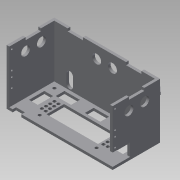
# Autodesk Inventor part: Kepala Belakang 2
Saved by Autodesk Inventor 2015 SP1 (Build 190203100, 203)
## iProperties
Created: 2015-02-01
Part Number: Kepala Belakang 2
Material: Generic
Document SubType Name: Modeling
Designer: Rafi Kurnia Putra
Density: 1 g/cm^3
Appearance: Default
Mass: 66.641 g
Surface Area: 406.742 cm^2
Volume: 66.641 cm^3
Author: Rafi Kurnia Putra
Autodesk Inventor part; units mm, degrees
(part 1 of 2)
ref_plane "YZ Plane" through (0, 0, 0) normal (1, 0, 0) x (0, 1, 0)
ref_plane "XY Plane" through (0, 0, 0) normal (0, 0, 1) x (1, 0, 0)
sketch "Sketch1" plane through (0, 0, 0) normal (0, 1, 0) x (-1, 0, 0)
  line L0 (60.406, -27.1071) -> (-60.406, -27.1071)
  line L1 (-60.406, -27.1071) -> (-60.406, 27.1071)
  line L2 (-60.406, 27.1071) -> (60.406, 27.1071)
  line L3 (60.406, 27.1071) -> (60.406, -27.1071)
  line L4 (60.406, -27.1071) -> (-60.406, 27.1071) construction
  line L5 (-60.406, -27.1071) -> (60.406, 27.1071) construction
  line L6 (-57.406, 24.1071) -> (-57.406, -27.1071)
  line L7 (57.406, -27.1071) -> (57.406, 24.1071)
  line L8 (57.406, 24.1071) -> (-57.406, 24.1071)
  point P0 (0, 0)
  point P1 (0, 0)
  dimension "d49" = 120.812
  dimension "d51" = 3
  dimension "d57" = 3
  dimension "d58" = 3
  dimension "d59" = 114.812
  dimension "d61" = 51.2141
  constraints: 18 end point, 3 midpoint, 3 parallel, 2 point on line, 1 horizontal, 1 perpendicular, 1 other
  measures "d49" distance of L1.end L2.end
  measures "d51" distance between parallel lines of L6 L1
  measures "d57" distance between parallel lines of L7 L3
  measures "d58" distance between parallel lines of L8 L2
  measures "d59" distance between parallel lines of L7 L6
  measures "d61" distance between parallel lines of L8 L0
extrude "Extrusion5" add sketch "Sketch1" against normal blind 3
extrude "Extrusion6" add sketch "Sketch1" along normal blind 60 contours L0 L7 L8 L6 L1 L2 L3
sketch "Sketch6" plane through (0, -3, 0) normal (0, -1, 0) x (1, 0, 0)
  circle A0 centre (-50.5965, 17.5471) radius 1.75
  circle A1 centre (50.5965, 17.5471) radius 1
  circle A2 centre (50.5965, 17.5471) radius 1.75
  circle A3 centre (-50.5965, 17.5471) radius 1.75
  point P0 (0, 0)
  dimension "d62" = 3.5
  constraints: 4 centre point, 2 coincident, 1 concentric, 4 other
  measures "d62" diameter of A2
extrude "Extrusion7" cut sketch "Sketch6" against normal up to next contours A0 | A1 | A2
sketch "Sketch7" plane through (0, -3, 0) normal (0, -1, 0) x (1, 0, 0)
  line L0 (-53.556, -8.4641) -> (-43.556, -8.4641)
  line L1 (-43.556, -8.4641) -> (-43.556, 9.0359)
  line L2 (-43.556, 9.0359) -> (-53.556, 9.0359)
  line L3 (-53.556, 9.0359) -> (-53.556, -8.4641)
  line L4 (-53.556, -8.4641) -> (-43.556, 9.0359) construction
  line L5 (-43.556, -8.4641) -> (-53.556, 9.0359) construction
  line L6 (53.556, -8.4641) -> (43.556, -8.4641)
  line L7 (43.556, -8.4641) -> (43.556, 9.0359)
  line L8 (43.556, 9.0359) -> (53.556, 9.0359)
  line L9 (53.556, 9.0359) -> (53.556, -8.4641)
  line L10 (53.556, -8.4641) -> (43.556, 9.0359) construction
  line L11 (43.556, -8.4641) -> (53.556, 9.0359) construction
  line L12 (-42.0848, 10.5071) -> (-24.5848, 10.5071)
  line L13 (-24.5848, 10.5071) -> (-24.5848, 20.5071)
  line L14 (-24.5848, 20.5071) -> (-42.0848, 20.5071)
  line L15 (-42.0848, 20.5071) -> (-42.0848, 10.5071)
  line L16 (-42.0848, 10.5071) -> (-24.5848, 20.5071) construction
  line L17 (-24.5848, 10.5071) -> (-42.0848, 20.5071) construction
  line L18 (42.0848, 10.5071) -> (24.5848, 10.5071)
  line L19 (24.5848, 10.5071) -> (24.5848, 20.5071)
  line L20 (24.5848, 20.5071) -> (42.0848, 20.5071)
  line L21 (42.0848, 20.5071) -> (42.0848, 10.5071)
  line L22 (42.0848, 10.5071) -> (24.5848, 20.5071) construction
  line L23 (24.5848, 10.5071) -> (42.0848, 20.5071) construction
  point P0 (0, 0)
  point P1 (-48.556, 0.2859)
  point P2 (-48.556, 0.2859)
  point P3 (48.556, 0.2859)
  point P4 (48.556, 0.2859)
  point P5 (-33.3348, 15.5071)
  point P6 (-33.3348, 15.5071)
  point P7 (33.3348, 15.5071)
  point P8 (33.3348, 15.5071)
  dimension "d65" = 10
  dimension "d66" = 17.5
  dimension "d69" = 10
  constraints: 48 end point, 10 midpoint, 4 parallel, 2 horizontal, 2 perpendicular
  measures "d65" distance of L2.end L1.end
  measures "d66" distance of L1.end L0.end
  measures "d69" distance of L13.end L12.end
extrude "Extrusion8" cut sketch "Sketch7" against normal up to next
sketch "Sketch9" plane through (0, 60, 0) normal (0, 1, 0) x (1, 0, 0)
  line L0 (60.406, 8.4641) -> (56.906, 8.4641)
  line L1 (56.906, -9.0359) -> (60.406, -9.0359)
  line L2 (60.406, 8.4641) -> (60.406, -9.0359)
  line L3 (56.906, -9.0359) -> (56.906, 8.4641)
  line L4 (42.0848, -23.8571) -> (42.0848, -27.3571)
  line L5 (42.0848, -27.3571) -> (24.5848, -27.3571)
  line L6 (24.5848, -23.8571) -> (42.0848, -23.8571)
  line L7 (24.5848, -23.8571) -> (24.5848, -27.3571)
  line L8 (0, 0) -> (0, -13)
  line L9 (-60.406, 8.4641) -> (-56.906, 8.4641)
  line L10 (-56.906, -9.0359) -> (-60.406, -9.0359)
  line L11 (-60.406, 8.4641) -> (-60.406, -9.0359)
  line L12 (-56.906, -9.0359) -> (-56.906, 8.4641)
  line L13 (-42.0848, -23.8571) -> (-42.0848, -27.3571)
  line L14 (-42.0848, -27.3571) -> (-24.5848, -27.3571)
  line L15 (-24.5848, -23.8571) -> (-42.0848, -23.8571)
  line L16 (-24.5848, -23.8571) -> (-24.5848, -27.3571)
  constraints: 34 end point, 8 symmetric about line, 2 vertical, 1 horizontal, 1 parallel
extrude "Extrusion9" cut sketch "Sketch9" against normal blind 3
sketch "Sketch10" plane through (0, -3, 0) normal (0, -1, 0) x (1, 0, 0)
  circle A0 centre (-32.4485, -17.4559) radius 1.75
  circle A1 centre (-37.593, 4.5441) radius 1.75
  circle A2 centre (32.4355, -17.4559) radius 1.75
  circle A3 centre (37.593, 4.5441) radius 1.75
  point P0 (0, 0)
  dimension "d84" = 22
  dimension "d85" = 22
  constraints: 4 centre point, 4 other
  measures "d84" vertical distance of A1.centre A0.centre
  measures "d85" vertical distance of A3.centre A2.centre
extrude "Extrusion10" cut sketch "Sketch10" against normal up to next
sketch "Sketch12" plane through (-60.406, -3, -27.1071) normal (-1, 0, 0) x (0, 0, 1)
  circle A0 centre (3, 59.0338) radius 1
  circle A1 centre (3, 38.0338) radius 1
  arc A2 (6.0857, 8.75) -> (6.7857, 8.05) centre (6.7857, 8.75) ccw
  arc A3 (13.0857, 8.05) -> (13.7857, 8.75) centre (13.0857, 8.75) ccw
  line L0 (13.0857, 8.05) -> (6.7857, 8.05)
  arc A4 (7.3007, 11.65) -> (6.9007, 11.25) centre (7.3007, 11.25) ccw
  arc A5 (12.9707, 11.25) -> (12.5707, 11.65) centre (12.5707, 11.25) ccw
  line L1 (7.3007, 11.25) -> (13.0857, 8.75) construction
  line L2 (13.0857, 8.75) -> (6.7857, 8.75) construction
  line L3 (6.7857, 8.75) -> (12.5707, 11.25) construction
  line L4 (2.4357, 5.1113) -> (17.4357, 5.1113)
  line L5 (17.4357, 5.1113) -> (17.4357, 15.1113)
  line L6 (17.4357, 15.1113) -> (2.4357, 15.1113)
  line L7 (2.4357, 15.1113) -> (2.4357, 5.1113)
  line L8 (2.4357, 5.1113) -> (17.4357, 15.1113) construction
  line L9 (17.4357, 5.1113) -> (2.4357, 15.1113) construction
  point P0 (27.1071, 3)
  point P1 (9.9357, 10.1113)
  dimension "d86" = 15
  dimension "d87" = 10
  constraints: 20 end point, 8 point on circle, 6 centre point, 3 horizontal, 2 midpoint, 2 parallel, 2 point on line, 1 perpendicular, 20 other
  measures "d86" distance of L6.end L5.end
  measures "d87" distance of L5.end L4.end
extrude "Extrusion11" cut sketch "Sketch12" against normal blind 200 contours A0 | A1
extrude "Extrusion12" cut sketch "Sketch12" against normal up to next contours L7 L6 L5 L4
fillet "Fillet2" radius 2 4 edges at (-58.906, 12.1113, -24.6713) (-58.906, 12.1113, -9.6713) (-58.906, 2.1113, -24.6713) (-58.906, 2.1113, -9.6713)
sketch "Sketch13" plane through (0, -3, 0) normal (0, -1, 0) x (1, 0, 0)
  line L0 (29.3575, 1.3171) -> (-29.3575, 1.3171)
  circle A0 centre (-32.8575, 4.3056) radius 1.75
  circle A1 centre (32.8575, 4.3056) radius 1.75
  line L1 (29.3575, 1.3171) -> (29.3575, 7.2941)
  line L2 (-29.3575, 1.3171) -> (-29.3575, 7.2941)
  line L3 (-29.3575, 7.2941) -> (29.3575, 7.2941)
  line L4 (-16, -57.1829) -> (-36, -57.1829)
  line L5 (-36, -57.1829) -> (-36, -2.1829)
  line L6 (-36, -2.1829) -> (-16, -2.1829)
  line L7 (-16, -2.1829) -> (-16, -57.1829)
  line L8 (-16, -57.1829) -> (-36, -2.1829) construction
  line L9 (-36, -57.1829) -> (-16, -2.1829) construction
  point P0 (0, 0)
  point P1 (34.6075, 4.3056)
  point P2 (29.3575, 4.3056)
  point P3 (-26, -29.6829)
  dimension "d96" = 3.5
  dimension "d95" = 3.5
  dimension "d97" = 3.5
  dimension "d99" = 20
  dimension "d100" = 55
  dimension "d101" = 3.5
  constraints: 20 end point, 3 horizontal, 3 perpendicular, 2 midpoint, 2 parallel, 1 centre point, 1 horizontal alignment, 3 other
  measures "d95" diameter of A0
  measures "d97" distance of point (32.857, 4.306) point (29.357, 4.306)
  measures "d99" distance of L5.end L6.end
  measures "d100" distance of L4.end L5.end
  measures "d101" distance between parallel lines of L0 L6
extrude "Extrusion13" cut sketch "Sketch13" against normal up to next contours L0 L2 L3 L1 | A0 | A1
ref_plane "Work Plane1" through (0, 19.75, 0) normal (0, 1, 0) x (-1, 0, 0)
sketch "Sketch20" plane through (-60.406, -3, -27.1071) normal (-1, 0, 0) x (0, 0, 1)
  line L0 (30.5999, 17.25) -> (30.5999, 19.25) projected
  arc A0 (31.0999, 19.75) -> (30.5999, 19.25) centre (31.0999, 19.25) ccw projected
  line L1 (31.0999, 19.75) -> (32.0999, 19.75) projected
  arc A1 (32.5999, 19.25) -> (32.0999, 19.75) centre (32.0999, 19.25) ccw projected
  line L2 (32.5999, 19.25) -> (32.5999, 17.25) projected
  line L3 (32.0999, 16.75) -> (31.0999, 16.75) projected
  arc A2 (30.5999, 17.25) -> (31.0999, 16.75) centre (31.0999, 17.25) ccw projected
  circle A3 centre (25.0999, 18.25) radius 3.75 projected
  arc A4 (32.0999, 16.75) -> (32.5999, 17.25) centre (32.0999, 17.25) ccw projected
  line L4 (31.0999, 19.25) -> (32.0999, 17.25) construction
  line L5 (32.0999, 17.25) -> (32.0999, 19.25) construction
  line L6 (30.5999, 19.25) -> (30.5999, 17.25) construction
  line L7 (32.0999, 19.25) -> (31.0999, 17.25) construction
  point P0 (27.1071, 3)
  point P1 (31.5999, 18.25)
  dimension "d132" = 6.5
  constraints: 6 end point, 1 midpoint, 1 parallel
  measures "d132" distance of point (31.6, 18.25) A3.centre
sketch "Sketch22" plane through (60.406, -3, 27.1071) normal (1, 0, 0) x (0, 0, -1)
  circle A0 centre (35.5712, 49.2838) radius 5.125
  circle A1 centre (17.5712, 49.2838) radius 5.125
  point P0 (27.1071, 3)
  point P1 (26.5712, 49.2838)
  dimension "d246" = 10.25
  dimension "d247" = 10.25
  dimension "d248" = 18
  dimension "d249" = 9
  constraints: 2 centre point, 1 other
  measures "d246" diameter of A0
  measures "d247" diameter of A1
  measures "d248" distance of A0.centre A1.centre
  measures "d249" distance of point (26.571, 49.284) A1.centre
sketch "Sketch23" plane through (-60.406, -3, 27.1071) normal (0, 0, 1) x (1, 0, 0)
  circle A0 centre (69.406, 49.2838) radius 5.125
  circle A1 centre (51.406, 49.2838) radius 5.125
  point P0 (60.406, 3)
  point P1 (60.406, 49.2838)
  dimension "d240" = 10.25
  dimension "d241" = 10.25
  dimension "d242" = 18
  dimension "d243" = 9
  constraints: 2 centre point, 1 other
  measures "d240" diameter of A0
  measures "d241" diameter of A1
  measures "d242" distance of A0.centre A1.centre
  measures "d243" distance of point (60.406, 49.284) A1.centre
sketch "Sketch24" plane through (0, -3, 0) normal (0, -1, 0) x (1, 0, 0)
  line L0 (53.556, -27.1071) -> (53.556, -43.2141)
  line L1 (43.556, -43.2141) -> (43.556, -27.1071)
  line L2 (53.556, -43.2141) -> (43.556, -43.2141)
  line L3 (53.556, -43.2141) -> (53.556, -23.2141)
  line L4 (53.556, -23.2141) -> (43.556, -23.2141)
  line L5 (43.556, -23.2141) -> (43.556, -27.1071)
  point P0 (0, 0)
  dimension "d164" = 20
  constraints: 12 end point, 3 vertical, 2 perpendicular, 1 horizontal, 4 other
  measures "d164" distance of L0.end L3.end
extrude "Extrusion26" cut sketch "Sketch24" against normal up to next
sketch "Sketch25" plane through (-60.406, -3, 27.1071) normal (0, 0, 1) x (1, 0, 0)
  line L0 (120.812, 22) -> (120.812, 14.5) projected
  line L1 (0, 63) -> (0, 0) projected
  line L2 (120.812, 18.25) -> (241.624, 18.25) construction
  circle A0 centre (41.322, 40.0298) radius 1.6 projected
  line L3 (41.322, 40.0298) -> (41.322, 18.25)
  circle A1 centre (79.49, 40.0298) radius 1.6 projected
  line L4 (79.49, 40.0298) -> (79.49, 18.25)
  line L5 (120.812, 18.25) -> (79.49, 18.25)
  line L6 (41.322, 18.25) -> (0, 18.25)
  arc A2 (103.901, 18.25) -> (96.401, 18.25) centre (100.151, 18.25) ccw
  arc A3 (24.411, 18.25) -> (16.911, 18.25) centre (20.661, 18.25) ccw
  arc A4 (16.911, 8) -> (24.411, 8) centre (20.661, 8) ccw
  arc A5 (96.401, 8) -> (103.901, 8) centre (100.151, 8) ccw
  line L7 (3, 3) -> (117.812, 3) projected
  line L8 (16.911, 18.25) -> (16.911, 8)
  line L9 (24.411, 18.25) -> (24.411, 8)
  line L10 (96.401, 18.25) -> (96.401, 8)
  line L11 (103.901, 18.25) -> (103.901, 8)
  point P0 (60.406, 3)
  dimension "d168" = 7.5
  dimension "d169" = 7.5
  dimension "d257" = 7.5
  dimension "d258" = 7.5
  dimension "d259" = 5
  dimension "d260" = 5
  constraints: 18 end point, 8 point on circle, 4 centre point, 4 perpendicular, 4 point on line, 4 tangent, 3 midpoint, 1 horizontal, 1 parallel
  measures "d168" diameter of A2
  measures "d169" diameter of A3
  measures "d257" diameter of A4
  measures "d258" diameter of A5
  measures "d259" distance from line of A4.centre L7
  measures "d260" distance from line of A5.centre L7
sketch "Sketch26" plane through (-60.406, -3, 27.1071) normal (0, 0, 1) x (1, 0, 0)
  circle A0 centre (20.661, 18.25) radius 3.75 projected
  circle A1 centre (100.151, 18.25) radius 3.75 projected
  line L0 (9.411, 40.5) -> (31.911, 40.5)
  line L1 (31.911, 40.5) -> (31.911, 37.5)
  line L2 (31.911, 37.5) -> (9.411, 37.5)
  line L3 (9.411, 37.5) -> (9.411, 40.5)
  line L4 (9.411, 40.5) -> (31.911, 37.5) construction
  line L5 (31.911, 40.5) -> (9.411, 37.5) construction
  line L6 (88.901, 40.5) -> (111.401, 40.5)
  line L7 (111.401, 40.5) -> (111.401, 37.5)
  line L8 (111.401, 37.5) -> (88.901, 37.5)
  line L9 (88.901, 37.5) -> (88.901, 40.5)
  line L10 (88.901, 40.5) -> (111.401, 37.5) construction
  line L11 (111.401, 40.5) -> (88.901, 37.5) construction
  line L12 (120.812, 0) -> (0, 0) projected
  point P0 (60.406, 3)
  point P1 (20.661, 39)
  point P2 (100.151, 39)
  dimension "d172" = 22.5
  dimension "d173" = 3
  dimension "d174" = 22.5
  dimension "d254" = 37.5
  dimension "d255" = 37.5
  dimension "d256" = 79.49
  constraints: 24 end point, 4 midpoint, 4 parallel, 2 horizontal, 2 perpendicular
  measures "d172" distance of L1.end L2.end
  measures "d173" distance of L0.end L1.end
  measures "d174" distance of L7.end L8.end
  measures "d254" distance between parallel lines of L12 L2
  measures "d255" distance between parallel lines of L12 L8
  measures "d256" distance of point (100.151, 39) point (20.661, 39)
extrude "Extrusion28" add sketch "Sketch26" along normal blind 15 contours L0 L1 L2 L3 | L6 L7 L8 L9
sketch "Sketch27" plane through (-50.995, 37.5, 27.1071) normal (0, 1, 0) x (1, 0, 0)
  circle A0 centre (-13.5951, 23.8524) radius 3.75 projected
  line L0 (0, 0) -> (22.5, 0) projected
  line L1 (0, 0) -> (0, -15) projected
  line L2 (22.5, -15) -> (0, -15) projected
  line L3 (22.5, 0) -> (22.5, -15) projected
  line L4 (79.49, 0) -> (101.99, 0) projected
  line L5 (79.49, 0) -> (79.49, -15) projected
  line L6 (101.99, -15) -> (79.49, -15) projected
  line L7 (101.99, 0) -> (101.99, -15) projected
  circle A1 centre (11.25, -7.5) radius 3.75
  circle A2 centre (90.74, -7.5) radius 3.75
  point P0 (50.995, 27.1071)
  dimension "d177" = 7.5
  dimension "d178" = 7.5
  constraints: 2 centre point
  measures "d177" diameter of A1
  measures "d178" diameter of A2
extrude "Extrusion29" cut sketch "Sketch27" against normal up to next contours A1 | A2
sketch "Sketch30" plane through (28.495, 37.5, 27.1071) normal (0, 1, 0) x (1, 0, 0)
  circle A0 centre (-68.24, -7.5) radius 3.75 projected
  circle A1 centre (11.25, -7.5) radius 3.75 projected
  line L0 (17.25, -9) -> (18.25, -9)
  line L1 (18.75, -8.5) -> (18.75, -6.5)
  line L2 (18.25, -6) -> (17.25, -6)
  line L3 (16.75, -6.5) -> (16.75, -8.5)
  line L4 (16.75, -9) -> (18.75, -6) construction
  line L5 (18.75, -9) -> (16.75, -6) construction
  line L6 (4.25, -9) -> (5.25, -9)
  line L7 (5.75, -8.5) -> (5.75, -6.5)
  line L8 (5.25, -6) -> (4.25, -6)
  line L9 (3.75, -6.5) -> (3.75, -8.5)
  line L10 (3.75, -9) -> (5.75, -6) construction
  line L11 (5.75, -9) -> (3.75, -6) construction
  line L12 (-62.24, -9) -> (-61.24, -9)
  line L13 (-60.74, -8.5) -> (-60.74, -6.5)
  line L14 (-61.24, -6) -> (-62.24, -6)
  line L15 (-62.74, -6.5) -> (-62.74, -8.5)
  line L16 (-62.74, -9) -> (-60.74, -6) construction
  line L17 (-60.74, -9) -> (-62.74, -6) construction
  line L18 (-74.24, -9) -> (-75.24, -9)
  line L19 (-75.74, -8.5) -> (-75.74, -6.5)
  line L20 (-75.24, -6) -> (-74.24, -6)
  line L21 (-73.74, -6.5) -> (-73.74, -8.5)
  line L22 (-73.74, -9) -> (-75.74, -6) construction
  line L23 (-75.74, -9) -> (-73.74, -6) construction
  arc A2 (-75.24, -6) -> (-75.74, -6.5) centre (-75.24, -6.5) ccw
  arc A3 (-73.74, -6.5) -> (-74.24, -6) centre (-74.24, -6.5) ccw
  arc A4 (-74.24, -9) -> (-73.74, -8.5) centre (-74.24, -8.5) ccw
  arc A5 (-75.74, -8.5) -> (-75.24, -9) centre (-75.24, -8.5) ccw
  arc A6 (-61.24, -9) -> (-60.74, -8.5) centre (-61.24, -8.5) ccw
  arc A7 (-60.74, -6.5) -> (-61.24, -6) centre (-61.24, -6.5) ccw
  arc A8 (-62.24, -6) -> (-62.74, -6.5) centre (-62.24, -6.5) ccw
  arc A9 (-62.74, -8.5) -> (-62.24, -9) centre (-62.24, -8.5) ccw
  arc A10 (16.75, -8.5) -> (17.25, -9) centre (17.25, -8.5) ccw
  arc A11 (17.25, -6) -> (16.75, -6.5) centre (17.25, -6.5) ccw
  arc A12 (18.75, -6.5) -> (18.25, -6) centre (18.25, -6.5) ccw
  arc A13 (18.25, -9) -> (18.75, -8.5) centre (18.25, -8.5) ccw
  arc A14 (5.25, -9) -> (5.75, -8.5) centre (5.25, -8.5) ccw
  arc A15 (5.75, -6.5) -> (5.25, -6) centre (5.25, -6.5) ccw
  arc A16 (4.25, -6) -> (3.75, -6.5) centre (4.25, -6.5) ccw
  arc A17 (3.75, -8.5) -> (4.25, -9) centre (4.25, -8.5) ccw
  point P0 (-28.495, 27.1071)
  point P1 (17.75, -7.5)
  point P2 (4.75, -7.5)
  point P3 (-61.74, -7.5)
  point P4 (-74.74, -7.5)
  dimension "d187" = 2
  dimension "d188" = 3
  dimension "d189" = 6.5
  dimension "d190" = 2
  dimension "d191" = 3
  dimension "d192" = 6.5
  dimension "d193" = 2
  dimension "d194" = 3
  dimension "d195" = 2
  dimension "d196" = 3
  dimension "d197" = 6.5
  dimension "d198" = 6.5
  dimension "d199" = 0.5
  constraints: 48 end point, 32 point on circle, 32 point on line, 32 tangent, 16 centre point, 15 equal radius, 8 midpoint, 8 parallel, 4 horizontal, 4 perpendicular
  measures "d187" distance of L5.end L4.end
  measures "d188" distance of L4.end L5.start
  measures "d189" distance of point (17.75, -7.5) A1.centre
  measures "d190" distance of L11.end L10.end
  measures "d191" distance of L10.end L11.start
  measures "d192" distance of point (4.75, -7.5) A1.centre
  measures "d193" distance of L17.end L16.end
  measures "d194" distance of L16.end L17.start
  measures "d195" distance of L22.end L23.end
  measures "d196" distance of L23.start L22.end
  measures "d197" distance of point (-74.74, -7.5) A0.centre
  measures "d198" distance of A0.centre point (-61.74, -7.5)
  measures "d199" radius of A2
extrude "Extrusion30" cut sketch "Sketch30" against normal up to next contours A10 L3 A11 L2 A12 L1 A13 L0 | A17 L9 A16 L8 A15 L7 A14 L6 | A9 L15 A8 L14 A7 L13 A6 L12 | L18 A5 L19 A2 L20 A3 L21 A4
chamfer "Chamfer1" distance 5 angle 45 4 edges at (-50.995, 36, 42.1071) (-28.495, 36, 42.1071) (28.495, 36, 42.1071) (50.995, 36, 42.1071)
sketch "Sketch34" plane through (-60.406, -3, -27.1071) normal (-1, 0, 0) x (0, 0, 1)
  line L0 (17.4357, 13.1113) -> (17.4357, 7.1113) projected
  arc A0 (15.4357, 5.1113) -> (17.4357, 7.1113) centre (15.4357, 7.1113) ccw projected
  line L1 (15.4357, 5.1113) -> (4.4357, 5.1113) projected
  arc A1 (2.4357, 7.1113) -> (4.4357, 5.1113) centre (4.4357, 7.1113) ccw projected
  line L2 (2.4357, 7.1113) -> (2.4357, 13.1113) projected
  arc A2 (4.4357, 15.1113) -> (2.4357, 13.1113) centre (4.4357, 13.1113) ccw projected
  line L3 (4.4357, 15.1113) -> (15.4357, 15.1113) projected
  arc A3 (17.4357, 13.1113) -> (15.4357, 15.1113) centre (15.4357, 13.1113) ccw projected
  circle A4 centre (3, 59.0338) radius 1 projected
  circle A5 centre (3, 38.0338) radius 1 projected
  line L4 (36.1429, 63) -> (36.1429, 60) projected
  line L5 (36.1429, 60) -> (18.6429, 60) projected
  line L6 (18.6429, 60) -> (18.6429, 63) projected
  line L7 (0, 63) -> (18.6429, 63) projected
  line L8 (0, 63) -> (0, 0) projected
  line L9 (54.2141, 0) -> (0, 0) projected
  line L10 (54.2141, 0) -> (54.2141, 63) projected
  line L11 (36.1429, 63) -> (54.2141, 63) projected
  line L12 (4.4357, 15.1113) -> (15.4357, 15.1113) projected
  arc A6 (4.4357, 15.1113) -> (2.4357, 13.1113) centre (4.4357, 13.1113) ccw projected
  line L13 (2.4357, 7.1113) -> (2.4357, 13.1113) projected
  arc A7 (2.4357, 7.1113) -> (4.4357, 5.1113) centre (4.4357, 7.1113) ccw projected
  line L14 (15.4357, 5.1113) -> (4.4357, 5.1113) projected
  arc A8 (15.4357, 5.1113) -> (17.4357, 7.1113) centre (15.4357, 7.1113) ccw projected
  line L15 (17.4357, 13.1113) -> (17.4357, 7.1113) projected
  arc A9 (17.4357, 13.1113) -> (15.4357, 15.1113) centre (15.4357, 13.1113) ccw projected
  line L16 (0, 3) -> (51.2141, 3) projected
  line L17 (19.8715, 17.2226) -> (0, 17.2226)
  line L18 (0, 17.2226) -> (0, 3)
  line L19 (0, 3) -> (19.8715, 3)
  line L20 (19.8715, 3) -> (19.8715, 17.2226)
  line L21 (19.8715, 17.2226) -> (0, 3) construction
  line L22 (0, 17.2226) -> (19.8715, 3) construction
  point P0 (27.1071, 3)
  point P1 (9.9357, 10.1113)
  constraints: 12 end point, 2 midpoint, 2 parallel, 1 horizontal, 1 perpendicular
extrude "Extrusion31" cut sketch "Sketch34" against normal blind 10 contours L0 A0 L1 A1 L2 A2 L3 A3 | L8 L17 L20 L16
sketch "Sketch35" plane through (0, 0, 0) normal (0, 1, 0) x (1, 0, 0)
  line L0 (-24.5848, -10.5071) -> (-24.5848, -20.5071) projected
  line L1 (-24.5848, -20.5071) -> (-42.0848, -20.5071) projected
  line L2 (-42.0848, -10.5071) -> (-24.5848, -10.5071) projected
  line L3 (-42.0848, -20.5071) -> (-42.0848, -10.5071) projected
  line L4 (-8.75, -10.5071) -> (8.75, -10.5071)
  line L5 (8.75, -10.5071) -> (8.75, -20.5071)
  line L6 (8.75, -20.5071) -> (-8.75, -20.5071)
  line L7 (-8.75, -20.5071) -> (-8.75, -10.5071)
  line L8 (-8.75, -10.5071) -> (8.75, -20.5071) construction
  line L9 (8.75, -10.5071) -> (-8.75, -20.5071) construction
  line L10 (29.3575, -1.3171) -> (29.3575, -7.2941) projected
  line L11 (-29.3575, -7.2941) -> (-29.3575, -1.3171) projected
  line L12 (29.3575, -1.3171) -> (-29.3575, -1.3171)
  line L13 (-29.3575, -1.3171) -> (-29.3575, 4.6829)
  line L14 (-29.3575, 4.6829) -> (29.3575, 4.6829)
  line L15 (29.3575, 4.6829) -> (29.3575, -1.3171)
  point P0 (0, 0)
  point P1 (0, -15.5071)
  dimension "d225" = 17.5
  dimension "d226" = 10
  dimension "d227" = 17.5
  dimension "d228" = 6
  constraints: 20 end point, 4 parallel, 2 horizontal, 2 midpoint, 2 perpendicular
  measures "d225" distance of L2.start L0.start
  measures "d226" distance between parallel lines of L2 L1
  measures "d227" distance of L5.end L6.end
  measures "d228" distance of L12.end L13.end
extrude "Extrusion32" cut sketch "Sketch35" against normal through all contours L4 L5 L6 L7 | L12 L13 L14 L15
extrude "Extrusion33" cut sketch "Sketch23" against normal up to next
extrude "Extrusion34" cut sketch "Sketch22" against normal through all
extrude "Extrusion35" cut sketch "Sketch25" against normal blind 10 contours L11 A5 L10 L5 | L5 A2 | L9 A4 L8 L6 | L6 A3
sketch "Sketch38" plane through (-60.406, -3, 27.1071) normal (0, 0, 1) x (1, 0, 0)
  line L0 (46.6835, 26.9535) -> (73.7901, 26.9535) construction
  line L1 (73.7901, 26.9535) -> (73.7901, 17.4497) construction
  line L2 (73.7901, 17.4497) -> (46.6835, 17.4497) construction
  line L3 (46.6835, 17.4497) -> (46.6835, 26.9535) construction
  line L4 (42.8938, 28.8402) -> (40.6025, 28.8402)
  line L5 (40.6025, 28.8402) -> (38.5178, 31.5935)
  line L6 (38.5178, 31.5935) -> (37.8371, 31.5935)
  line L7 (37.8371, 31.5935) -> (37.8371, 28.8402)
  line L8 (37.8371, 28.8402) -> (35.9651, 28.8402)
  line L9 (35.9651, 28.8402) -> (35.9651, 36.3402)
  line L10 (35.9651, 36.3402) -> (38.9797, 36.3402)
  spline S0 degree 2 poles (38.9797, 36.3402) (39.6057, 36.3402) (40.5296, 36.1822) (40.9246, 35.9391) knots 0 0 0 1 2 2 2
  spline S1 degree 2 poles (40.9246, 35.9391) (41.3257, 35.6838) (41.7998, 34.8876) (41.7998, 34.2799) knots 0 0 0 1 2 2 2
  spline S2 degree 2 poles (41.7998, 34.2799) (41.7998, 33.4229) (41.0219, 32.3471) (40.3715, 32.0311) knots 0 0 0 1 2 2 2
  line L11 (40.3715, 32.0311) -> (42.8938, 28.8402)
  spline S3 degree 2 poles (39.8671, 34.0428) (39.8671, 34.3285) (39.6483, 34.7357) (39.3991, 34.8451) knots 0 0 0 1 2 2 2
  spline S4 degree 2 poles (39.3991, 34.8451) (39.2228, 34.918) (38.7913, 34.9606) (38.4692, 34.9606) knots 0 0 0 1 2 2 2
  line L12 (38.4692, 34.9606) -> (37.8371, 34.9606)
  line L13 (37.8371, 34.9606) -> (37.8371, 32.9427)
  line L14 (37.8371, 32.9427) -> (38.378, 32.9427)
  spline S5 degree 2 poles (38.378, 32.9427) (38.767, 32.9427) (39.3201, 33.04) (39.5085, 33.1919) knots 0 0 0 1 2 2 2
  spline S6 degree 2 poles (39.5085, 33.1919) (39.6908, 33.3378) (39.8671, 33.7268) (39.8671, 34.0428) knots 0 0 0 1 2 2 2
  spline S7 degree 2 poles (50.2783, 32.5902) (50.2783, 30.7669) (48.3334, 28.6822) (46.6438, 28.6822) knots 0 0 0 1 2 2 2
  spline S8 degree 2 poles (46.6438, 28.6822) (44.9481, 28.6822) (43.0154, 30.7912) (43.0154, 32.5902) knots 0 0 0 1 2 2 2
  spline S9 degree 2 poles (43.0154, 32.5902) (43.0154, 34.3953) (44.9481, 36.4982) (46.6438, 36.4982) knots 0 0 0 1 2 2 2
  spline S10 degree 2 poles (46.6438, 36.4982) (48.3334, 36.4982) (50.2783, 34.4075) (50.2783, 32.5902) knots 0 0 0 1 2 2 2
  spline S11 degree 2 poles (48.3334, 32.5902) (48.3334, 33.2649) (48.0599, 34.2069) (47.8229, 34.5047) knots 0 0 0 1 2 2 2
  spline S12 degree 2 poles (47.8229, 34.5047) (47.5859, 34.8147) (46.9781, 35.0821) (46.6499, 35.0821) knots 0 0 0 1 2 2 2
  spline S13 degree 2 poles (46.6499, 35.0821) (46.3035, 35.0821) (45.7382, 34.8329) (45.4769, 34.5169) knots 0 0 0 1 2 2 2
  spline S14 degree 2 poles (45.4769, 34.5169) (45.2459, 34.2252) (44.9603, 33.2588) (44.9603, 32.5902) knots 0 0 0 1 2 2 2
  spline S15 degree 2 poles (44.9603, 32.5902) (44.9603, 31.8974) (45.2338, 30.9857) (45.4708, 30.6757) knots 0 0 0 1 2 2 2
  spline S16 degree 2 poles (45.4708, 30.6757) (45.7078, 30.3658) (46.3217, 30.0983) (46.6499, 30.0983) knots 0 0 0 1 2 2 2
  spline S17 degree 2 poles (46.6499, 30.0983) (46.9842, 30.0983) (47.6041, 30.384) (47.829, 30.6879) knots 0 0 0 1 2 2 2
  spline S18 degree 2 poles (47.829, 30.6879) (48.0721, 31.0161) (48.3334, 31.8852) (48.3334, 32.5902) knots 0 0 0 1 2 2 2
  spline S19 degree 2 poles (57.3894, 31.1376) (57.3894, 30.5785) (56.9639, 29.7337) (56.6114, 29.4541) knots 0 0 0 1 2 2 2
  spline S20 degree 2 poles (56.6114, 29.4541) (56.186, 29.1198) (55.177, 28.8402) (54.393, 28.8402) knots 0 0 0 1 2 2 2
  line L15 (54.393, 28.8402) -> (51.3967, 28.8402)
  line L16 (51.3967, 28.8402) -> (51.3967, 36.3402)
  line L17 (51.3967, 36.3402) -> (54.0405, 36.3402)
  spline S21 degree 2 poles (54.0405, 36.3402) (54.8671, 36.3402) (55.718, 36.2126) (56.0887, 36.012) knots 0 0 0 1 2 2 2
  spline S22 degree 2 poles (56.0887, 36.012) (56.4959, 35.7993) (56.891, 35.07) (56.891, 34.5959) knots 0 0 0 1 2 2 2
  spline S23 degree 2 poles (56.891, 34.5959) (56.891, 34.0489) (56.344, 33.1919) (55.8578, 32.9914) knots 0 0 0 1 2 2 2
  line L18 (55.8578, 32.9914) -> (55.8578, 32.9549)
  spline S24 degree 2 poles (55.8578, 32.9549) (56.5567, 32.809) (57.3894, 31.9034) (57.3894, 31.1376) knots 0 0 0 1 2 2 2
  spline S25 degree 2 poles (55.4445, 31.168) (55.4445, 31.5205) (55.1649, 31.9156) (54.8853, 32.0189) knots 0 0 0 1 2 2 2
  spline S26 degree 2 poles (54.8853, 32.0189) (54.7151, 32.0858) (54.1134, 32.0979) (53.6151, 32.0979) knots 0 0 0 1 2 2 2
  line L19 (53.6151, 32.0979) -> (53.2686, 32.0979)
  line L20 (53.2686, 32.0979) -> (53.2686, 30.2077)
  line L21 (53.2686, 30.2077) -> (53.3719, 30.2077)
  spline S27 degree 2 poles (53.3719, 30.2077) (54.1013, 30.2077) (54.6604, 30.226) (54.9522, 30.3536) knots 0 0 0 1 2 2 2
  spline S28 degree 2 poles (54.9522, 30.3536) (55.2074, 30.4691) (55.4445, 30.8945) (55.4445, 31.168) knots 0 0 0 1 2 2 2
  spline S29 degree 2 poles (54.9765, 34.2252) (54.9765, 34.4075) (54.7881, 34.7904) (54.5936, 34.8755) knots 0 0 0 1 2 2 2
  spline S30 degree 2 poles (54.5936, 34.8755) (54.4112, 34.9606) (53.9007, 34.9727) (53.3962, 34.9727) knots 0 0 0 1 2 2 2
  line L22 (53.3962, 34.9727) -> (53.2686, 34.9727)
  line L23 (53.2686, 34.9727) -> (53.2686, 33.3803)
  line L24 (53.2686, 33.3803) -> (53.5057, 33.3803)
  spline S31 degree 2 poles (53.5057, 33.3803) (53.9858, 33.3803) (54.3748, 33.3986) (54.5814, 33.4958) knots 0 0 0 1 2 2 2
  spline S32 degree 2 poles (54.5814, 33.4958) (54.8063, 33.6052) (54.9765, 33.976) (54.9765, 34.2252) knots 0 0 0 1 2 2 2
  spline S33 degree 2 poles (61.504, 28.6822) (59.9907, 28.6822) (58.3618, 30.1409) (58.3618, 31.5509) knots 0 0 0 1 2 2 2
  line L25 (58.3618, 31.5509) -> (58.3618, 36.3402)
  line L26 (58.3618, 36.3402) -> (60.2459, 36.3402)
  line L27 (60.2459, 36.3402) -> (60.2459, 31.6603)
  spline S34 degree 2 poles (60.2459, 31.6603) (60.2459, 30.8763) (60.8355, 30.1105) (61.504, 30.1105) knots 0 0 0 1 2 2 2
  spline S35 degree 2 poles (61.504, 30.1105) (62.1544, 30.1105) (62.7621, 30.8459) (62.7621, 31.6603) knots 0 0 0 1 2 2 2
  line L28 (62.7621, 31.6603) -> (62.7621, 36.3402)
  line L29 (62.7621, 36.3402) -> (64.6462, 36.3402)
  line L30 (64.6462, 36.3402) -> (64.6462, 31.557)
  spline S36 degree 2 poles (64.6462, 31.557) (64.6462, 30.1713) (63.0599, 28.6822) (61.504, 28.6822) knots 0 0 0 1 2 2 2
  spline S37 degree 2 poles (68.4084, 28.7065) (67.5454, 28.7065) (66.2447, 29.0408) (65.6856, 29.2839) knots 0 0 0 1 2 2 2
  line L31 (65.6856, 29.2839) -> (65.6856, 31.0708)
  line L32 (65.6856, 31.0708) -> (65.8557, 31.0708)
  spline S38 degree 2 poles (65.8557, 31.0708) (66.421, 30.5906) (67.7763, 30.074) (68.4145, 30.074) knots 0 0 0 1 2 2 2
  spline S39 degree 2 poles (68.4145, 30.074) (68.5786, 30.074) (69.1074, 30.147) (69.2654, 30.2199) knots 0 0 0 1 2 2 2
  spline S40 degree 2 poles (69.2654, 30.2199) (69.4599, 30.305) (69.7334, 30.6149) (69.7334, 30.8641) knots 0 0 0 1 2 2 2
  spline S41 degree 2 poles (69.7334, 30.8641) (69.7334, 31.1498) (69.2897, 31.5023) (68.9858, 31.5813) knots 0 0 0 1 2 2 2
  spline S42 degree 2 poles (68.9858, 31.5813) (68.6029, 31.6846) (67.7338, 31.8609) (67.3509, 31.9946) knots 0 0 0 1 2 2 2
  spline S43 degree 2 poles (67.3509, 31.9946) (66.4817, 32.2985) (65.7281, 33.3378) (65.7281, 34.1158) knots 0 0 0 1 2 2 2
  spline S44 degree 2 poles (65.7281, 34.1158) (65.7281, 35.1672) (67.5089, 36.4739) (68.846, 36.4739) knots 0 0 0 1 2 2 2
  spline S45 degree 2 poles (68.846, 36.4739) (69.5146, 36.4739) (70.8395, 36.2004) (71.3622, 35.9695) knots 0 0 0 1 2 2 2
  line L33 (71.3622, 35.9695) -> (71.3622, 34.2555)
  line L34 (71.3622, 34.2555) -> (71.1981, 34.2555)
  spline S46 degree 2 poles (71.1981, 34.2555) (70.7787, 34.6141) (69.5753, 35.1064) (68.9433, 35.1064) knots 0 0 0 1 2 2 2
  spline S47 degree 2 poles (68.9433, 35.1064) (68.6941, 35.1064) (68.3051, 35.0335) (68.0863, 34.9363) knots 0 0 0 1 2 2 2
  spline S48 degree 2 poles (68.0863, 34.9363) (67.91, 34.8572) (67.6548, 34.5412) (67.6548, 34.3467) knots 0 0 0 1 2 2 2
  spline S49 degree 2 poles (67.6548, 34.3467) (67.6548, 34.055) (68.062, 33.7207) (68.6454, 33.587) knots 0 0 0 1 2 2 2
  spline S50 degree 2 poles (68.6454, 33.587) (69.0223, 33.5019) (69.7212, 33.3378) (70.1223, 33.198) knots 0 0 0 1 2 2 2
  spline S51 degree 2 poles (70.1223, 33.198) (70.9003, 32.9124) (71.66, 31.9642) (71.66, 31.1863) knots 0 0 0 1 2 2 2
  spline S52 degree 2 poles (71.66, 31.1863) (71.66, 30.0679) (69.9035, 28.7065) (68.4084, 28.7065) knots 0 0 0 1 2 2 2
  line L35 (74.0668, 28.8402) -> (74.0668, 34.9119)
  line L36 (74.0668, 34.9119) -> (71.8484, 34.9119)
  line L37 (71.8484, 34.9119) -> (71.8484, 36.3402)
  line L38 (71.8484, 36.3402) -> (78.1693, 36.3402)
  line L39 (78.1693, 36.3402) -> (78.1693, 34.9119)
  line L40 (78.1693, 34.9119) -> (75.951, 34.9119)
  line L41 (75.951, 34.9119) -> (75.951, 28.8402)
  line L42 (75.951, 28.8402) -> (74.0668, 28.8402)
  line L43 (78.1329, 28.8402) -> (80.6673, 36.3402)
  line L44 (80.6673, 36.3402) -> (82.7216, 36.3402)
  line L45 (82.7216, 36.3402) -> (85.2561, 28.8402)
  line L46 (85.2561, 28.8402) -> (83.3172, 28.8402)
  line L47 (83.3172, 28.8402) -> (82.8492, 30.3718)
  line L48 (82.8492, 30.3718) -> (80.4911, 30.3718)
  line L49 (80.4911, 30.3718) -> (80.017, 28.8402)
  line L50 (80.017, 28.8402) -> (78.1329, 28.8402)
  line L51 (82.436, 31.7333) -> (81.6702, 34.213)
  line L52 (81.6702, 34.213) -> (80.8983, 31.7333)
  line L53 (80.8983, 31.7333) -> (82.436, 31.7333)
  spline S53 degree 2 poles (39.7148, 17.9633) (38.4839, 17.9633) (37.1591, 19.1497) (37.1591, 20.2965) knots 0 0 0 1 2 2 2
  line L54 (37.1591, 20.2965) -> (37.1591, 24.1918)
  line L55 (37.1591, 24.1918) -> (38.6915, 24.1918)
  line L56 (38.6915, 24.1918) -> (38.6915, 20.3855)
  spline S54 degree 2 poles (38.6915, 20.3855) (38.6915, 19.7478) (39.171, 19.125) (39.7148, 19.125) knots 0 0 0 1 2 2 2
  spline S55 degree 2 poles (39.7148, 19.125) (40.2437, 19.125) (40.7381, 19.7231) (40.7381, 20.3855) knots 0 0 0 1 2 2 2
  line L57 (40.7381, 20.3855) -> (40.7381, 24.1918)
  line L58 (40.7381, 24.1918) -> (42.2705, 24.1918)
  line L59 (42.2705, 24.1918) -> (42.2705, 20.3015)
  spline S56 degree 2 poles (42.2705, 20.3015) (42.2705, 19.1744) (40.9803, 17.9633) (39.7148, 17.9633) knots 0 0 0 1 2 2 2
  line L60 (47.6685, 18.0918) -> (46.2251, 18.0918)
  line L61 (46.2251, 18.0918) -> (46.2251, 20.3707)
  spline S57 degree 2 poles (46.2251, 20.3707) (46.2251, 20.6525) (46.1806, 21.2061) (46.1213, 21.3346) knots 0 0 0 1 2 2 2
  spline S58 degree 2 poles (46.1213, 21.3346) (46.0471, 21.4928) (45.7703, 21.6263) (45.533, 21.6263) knots 0 0 0 1 2 2 2
  spline S59 degree 2 poles (45.533, 21.6263) (45.36, 21.6263) (44.9992, 21.4928) (44.7965, 21.3495) knots 0 0 0 1 2 2 2
  line L62 (44.7965, 21.3495) -> (44.7965, 18.0918)
  line L63 (44.7965, 18.0918) -> (43.3629, 18.0918)
  line L64 (43.3629, 18.0918) -> (43.3629, 22.694)
  line L65 (43.3629, 22.694) -> (44.7965, 22.694)
  line L66 (44.7965, 22.694) -> (44.7965, 22.1849)
  spline S60 degree 2 poles (44.7965, 22.1849) (45.1475, 22.4815) (45.8148, 22.8176) (46.2202, 22.8176) knots 0 0 0 1 2 2 2
  spline S61 degree 2 poles (46.2202, 22.8176) (46.9221, 22.8176) (47.6685, 21.9278) (47.6685, 21.0875) knots 0 0 0 1 2 2 2
  line L67 (47.6685, 21.0875) -> (47.6685, 18.0918)
  line L68 (50.1649, 18.0918) -> (48.7313, 18.0918)
  line L69 (48.7313, 18.0918) -> (48.7313, 22.694)
  line L70 (48.7313, 22.694) -> (50.1649, 22.694)
  line L71 (50.1649, 22.694) -> (50.1649, 18.0918)
  line L72 (50.2094, 23.3515) -> (48.6918, 23.3515)
  line L73 (48.6918, 23.3515) -> (48.6918, 24.4687)
  line L74 (48.6918, 24.4687) -> (50.2094, 24.4687)
  line L75 (50.2094, 24.4687) -> (50.2094, 23.3515)
  line L76 (55.5679, 22.694) -> (53.9168, 18.0918)
  line L77 (53.9168, 18.0918) -> (52.3498, 18.0918)
  line L78 (52.3498, 18.0918) -> (50.7136, 22.694)
  line L79 (50.7136, 22.694) -> (52.2213, 22.694)
  line L80 (52.2213, 22.694) -> (53.1605, 19.6539)
  line L81 (53.1605, 19.6539) -> (54.0898, 22.694)
  line L82 (54.0898, 22.694) -> (55.5679, 22.694)
  spline S62 degree 2 poles (58.4745, 17.9683) (57.1695, 17.9683) (55.7804, 19.214) (55.7804, 20.3657) knots 0 0 0 1 2 2 2
  spline S63 degree 2 poles (55.7804, 20.3657) (55.7804, 21.4928) (57.0756, 22.8374) (58.2422, 22.8374) knots 0 0 0 1 2 2 2
  spline S64 degree 2 poles (58.2422, 22.8374) (59.2951, 22.8374) (60.3629, 21.6955) (60.3629, 20.6376) knots 0 0 0 1 2 2 2
  line L83 (60.3629, 20.6376) -> (60.3629, 20.1186)
  line L84 (60.3629, 20.1186) -> (57.214, 20.1186)
  spline S65 degree 2 poles (57.214, 20.1186) (57.2338, 19.7973) (57.4661, 19.3721) (57.6539, 19.2436) knots 0 0 0 1 2 2 2
  spline S66 degree 2 poles (57.6539, 19.2436) (57.8369, 19.1151) (58.3312, 19.0063) (58.6228, 19.0063) knots 0 0 0 1 2 2 2
  spline S67 degree 2 poles (58.6228, 19.0063) (58.87, 19.0063) (59.3544, 19.1151) (59.5571, 19.209) knots 0 0 0 1 2 2 2
  spline S68 degree 2 poles (59.5571, 19.209) (59.7351, 19.2832) (60.0317, 19.4661) (60.1256, 19.5353) knots 0 0 0 1 2 2 2
  line L85 (60.1256, 19.5353) -> (60.2788, 19.5353)
  line L86 (60.2788, 19.5353) -> (60.2788, 18.3489)
  spline S69 degree 2 poles (60.2788, 18.3489) (60.1009, 18.2797) (59.8142, 18.161) (59.5571, 18.1017) knots 0 0 0 1 2 2 2
  spline S70 degree 2 poles (59.5571, 18.1017) (59.3248, 18.0375) (58.8304, 17.9683) (58.4745, 17.9683) knots 0 0 0 1 2 2 2
  spline S71 degree 2 poles (58.9491, 20.9837) (58.9392, 21.4384) (58.5388, 21.9179) (58.1285, 21.9179) knots 0 0 0 1 2 2 2
  spline S72 degree 2 poles (58.1285, 21.9179) (57.7083, 21.9179) (57.2338, 21.4137) (57.2091, 20.9837) knots 0 0 0 1 2 2 2
  line L87 (57.2091, 20.9837) -> (58.9491, 20.9837)
  line L88 (64.189, 21.3346) -> (64.0703, 21.3346)
  spline S73 degree 2 poles (64.0703, 21.3346) (63.9863, 21.3643) (63.6749, 21.3939) (63.487, 21.3939) knots 0 0 0 1 2 2 2
  spline S74 degree 2 poles (63.487, 21.3939) (63.2646, 21.3939) (62.7653, 21.2605) (62.533, 21.1715) knots 0 0 0 1 2 2 2
  line L89 (62.533, 21.1715) -> (62.533, 18.0918)
  line L90 (62.533, 18.0918) -> (61.0994, 18.0918)
  line L91 (61.0994, 18.0918) -> (61.0994, 22.694)
  line L92 (61.0994, 22.694) -> (62.533, 22.694)
  line L93 (62.533, 22.694) -> (62.533, 22.0316)
  spline S75 degree 2 poles (62.533, 22.0316) (62.6318, 22.1206) (62.9779, 22.3974) (63.1212, 22.4815) knots 0 0 0 1 2 2 2
  spline S76 degree 2 poles (63.1212, 22.4815) (63.2794, 22.5754) (63.6946, 22.7089) (63.8775, 22.7089) knots 0 0 0 1 2 2 2
  spline S77 degree 2 poles (63.8775, 22.7089) (63.9467, 22.7089) (64.1198, 22.699) (64.189, 22.694) knots 0 0 0 1 2 2 2
  line L94 (64.189, 22.694) -> (64.189, 21.3346)
  spline S78 degree 2 poles (66.1366, 17.9683) (65.6324, 17.9683) (64.7278, 18.1907) (64.4312, 18.339) knots 0 0 0 1 2 2 2
  line L95 (64.4312, 18.339) -> (64.4312, 19.5501)
  line L96 (64.4312, 19.5501) -> (64.5498, 19.5501)
  spline S79 degree 2 poles (64.5498, 19.5501) (64.6536, 19.471) (64.9156, 19.2832) (65.148, 19.1794) knots 0 0 0 1 2 2 2
  spline S80 degree 2 poles (65.148, 19.1794) (65.3506, 19.0854) (65.8499, 18.952) (66.1465, 18.952) knots 0 0 0 1 2 2 2
  spline S81 degree 2 poles (66.1465, 18.952) (66.448, 18.952) (66.9127, 19.1398) (66.9127, 19.3425) knots 0 0 0 1 2 2 2
  spline S82 degree 2 poles (66.9127, 19.3425) (66.9127, 19.5007) (66.7001, 19.6687) (66.3937, 19.7379) knots 0 0 0 1 2 2 2
  spline S83 degree 2 poles (66.3937, 19.7379) (66.2305, 19.7824) (65.7313, 19.8764) (65.5385, 19.9357) knots 0 0 0 1 2 2 2
  spline S84 degree 2 poles (65.5385, 19.9357) (64.9947, 20.1038) (64.451, 20.7612) (64.451, 21.3) knots 0 0 0 1 2 2 2
  spline S85 degree 2 poles (64.451, 21.3) (64.451, 21.6065) (64.7327, 22.1503) (65.0095, 22.3628) knots 0 0 0 1 2 2 2
  spline S86 degree 2 poles (65.0095, 22.3628) (65.2814, 22.5704) (66.0872, 22.8176) (66.5963, 22.8176) knots 0 0 0 1 2 2 2
  spline S87 degree 2 poles (66.5963, 22.8176) (67.0808, 22.8176) (67.8915, 22.6248) (68.1683, 22.4914) knots 0 0 0 1 2 2 2
  line L97 (68.1683, 22.4914) -> (68.1683, 21.3247)
  line L98 (68.1683, 21.3247) -> (68.0546, 21.3247)
  spline S88 degree 2 poles (68.0546, 21.3247) (67.9804, 21.3841) (67.6591, 21.5768) (67.5108, 21.6461) knots 0 0 0 1 2 2 2
  spline S89 degree 2 poles (67.5108, 21.6461) (67.3279, 21.7251) (66.883, 21.8339) (66.6507, 21.8339) knots 0 0 0 1 2 2 2
  spline S90 degree 2 poles (66.6507, 21.8339) (66.3393, 21.8339) (65.9092, 21.6213) (65.9092, 21.4483) knots 0 0 0 1 2 2 2
  spline S91 degree 2 poles (65.9092, 21.4483) (65.9092, 21.2901) (66.1218, 21.1122) (66.4777, 21.0232) knots 0 0 0 1 2 2 2
  spline S92 degree 2 poles (66.4777, 21.0232) (66.6606, 20.9787) (67.1401, 20.8947) (67.3625, 20.8205) knots 0 0 0 1 2 2 2
  spline S93 degree 2 poles (67.3625, 20.8205) (67.8569, 20.6623) (68.371, 20.0444) (68.371, 19.5303) knots 0 0 0 1 2 2 2
  spline S94 degree 2 poles (68.371, 19.5303) (68.371, 19.209) (68.0694, 18.6208) (67.7877, 18.423) knots 0 0 0 1 2 2 2
  spline S95 degree 2 poles (67.7877, 18.423) (67.496, 18.2055) (66.6952, 17.9683) (66.1366, 17.9683) knots 0 0 0 1 2 2 2
  line L99 (70.4867, 18.0918) -> (69.0531, 18.0918)
  line L100 (69.0531, 18.0918) -> (69.0531, 22.694)
  line L101 (69.0531, 22.694) -> (70.4867, 22.694)
  line L102 (70.4867, 22.694) -> (70.4867, 18.0918)
  line L103 (70.5312, 23.3515) -> (69.0136, 23.3515)
  line L104 (69.0136, 23.3515) -> (69.0136, 24.4687)
  line L105 (69.0136, 24.4687) -> (70.5312, 24.4687)
  line L106 (70.5312, 24.4687) -> (70.5312, 23.3515)
  spline S96 degree 2 poles (73.3439, 18.0029) (72.4689, 18.0029) (71.6681, 18.7246) (71.6681, 19.5452) knots 0 0 0 1 2 2 2
  line L107 (71.6681, 19.5452) -> (71.6681, 21.6955)
  line L108 (71.6681, 21.6955) -> (71.1194, 21.6955)
  line L109 (71.1194, 21.6955) -> (71.1194, 22.694)
  line L110 (71.1194, 22.694) -> (71.6681, 22.694)
  line L111 (71.6681, 22.694) -> (71.6681, 24.0089)
  line L112 (71.6681, 24.0089) -> (73.1017, 24.0089)
  line L113 (73.1017, 24.0089) -> (73.1017, 22.694)
  line L114 (73.1017, 22.694) -> (74.4858, 22.694)
  line L115 (74.4858, 22.694) -> (74.4858, 21.6955)
  line L116 (74.4858, 21.6955) -> (73.1017, 21.6955)
  line L117 (73.1017, 21.6955) -> (73.1017, 20.0593)
  spline S97 degree 2 poles (73.1017, 20.0593) (73.1017, 19.817) (73.1116, 19.4562) (73.1709, 19.3128) knots 0 0 0 1 2 2 2
  spline S98 degree 2 poles (73.1709, 19.3128) (73.2302, 19.1695) (73.5219, 19.0014) (73.7987, 19.0014) knots 0 0 0 1 2 2 2
  spline S99 degree 2 poles (73.7987, 19.0014) (73.9173, 19.0014) (74.2881, 19.1003) (74.3622, 19.1398) knots 0 0 0 1 2 2 2
  line L118 (74.3622, 19.1398) -> (74.4858, 19.1398)
  line L119 (74.4858, 19.1398) -> (74.4858, 18.1314)
  spline S100 degree 2 poles (74.4858, 18.1314) (74.2535, 18.0721) (73.7295, 18.0029) (73.3439, 18.0029) knots 0 0 0 1 2 2 2
  spline S101 degree 2 poles (77.605, 18.5812) (77.4567, 18.4576) (77.2244, 18.2599) (77.0266, 18.161) knots 0 0 0 1 2 2 2
  spline S102 degree 2 poles (77.0266, 18.161) (76.8339, 18.0671) (76.4681, 17.9683) (76.1418, 17.9683) knots 0 0 0 1 2 2 2
  spline S103 degree 2 poles (76.1418, 17.9683) (75.5288, 17.9683) (74.7231, 18.7888) (74.7231, 19.4117) knots 0 0 0 1 2 2 2
  spline S104 degree 2 poles (74.7231, 19.4117) (74.7231, 19.9208) (75.1334, 20.5536) (75.5189, 20.7365) knots 0 0 0 1 2 2 2
  spline S105 degree 2 poles (75.5189, 20.7365) (75.9095, 20.9243) (76.992, 21.0726) (77.6149, 21.1122) knots 0 0 0 1 2 2 2
  line L120 (77.6149, 21.1122) -> (77.6149, 21.1369)
  spline S106 degree 2 poles (77.6149, 21.1369) (77.6149, 21.5175) (77.0514, 21.8092) (76.4878, 21.8092) knots 0 0 0 1 2 2 2
  spline S107 degree 2 poles (76.4878, 21.8092) (76.2357, 21.8092) (75.5535, 21.6263) (75.2322, 21.4829) knots 0 0 0 1 2 2 2
  line L121 (75.2322, 21.4829) -> (75.1086, 21.4829)
  line L122 (75.1086, 21.4829) -> (75.1086, 22.5952)
  spline S108 degree 2 poles (75.1086, 22.5952) (75.3212, 22.6545) (76.2703, 22.8226) (76.7548, 22.8226) knots 0 0 0 1 2 2 2
  spline S109 degree 2 poles (76.7548, 22.8226) (77.9411, 22.8226) (79.0287, 22.0316) (79.0287, 21.2209) knots 0 0 0 1 2 2 2
  line L123 (79.0287, 21.2209) -> (79.0287, 18.0918)
  line L124 (79.0287, 18.0918) -> (77.605, 18.0918)
  line L125 (77.605, 18.0918) -> (77.605, 18.5812)
  line L126 (77.605, 19.2931) -> (77.605, 20.2471)
  spline S110 degree 2 poles (77.605, 20.2471) (77.2392, 20.2125) (76.7894, 20.1581) (76.5719, 20.079) knots 0 0 0 1 2 2 2
  spline S111 degree 2 poles (76.5719, 20.079) (76.3791, 20.0148) (76.1715, 19.7478) (76.1715, 19.5303) knots 0 0 0 1 2 2 2
  spline S112 degree 2 poles (76.1715, 19.5303) (76.1715, 19.209) (76.5224, 18.9668) (76.8635, 18.9668) knots 0 0 0 1 2 2 2
  spline S113 degree 2 poles (76.8635, 18.9668) (77.0514, 18.9668) (77.4468, 19.1398) (77.605, 19.2931) knots 0 0 0 1 2 2 2
  spline S114 degree 2 poles (81.4904, 17.9683) (80.9862, 17.9683) (80.0816, 18.1907) (79.785, 18.339) knots 0 0 0 1 2 2 2
  line L127 (79.785, 18.339) -> (79.785, 19.5501)
  line L128 (79.785, 19.5501) -> (79.9036, 19.5501)
  spline S115 degree 2 poles (79.9036, 19.5501) (80.0074, 19.471) (80.2694, 19.2832) (80.5018, 19.1794) knots 0 0 0 1 2 2 2
  spline S116 degree 2 poles (80.5018, 19.1794) (80.7044, 19.0854) (81.2037, 18.952) (81.5003, 18.952) knots 0 0 0 1 2 2 2
  spline S117 degree 2 poles (81.5003, 18.952) (81.8018, 18.952) (82.2665, 19.1398) (82.2665, 19.3425) knots 0 0 0 1 2 2 2
  spline S118 degree 2 poles (82.2665, 19.3425) (82.2665, 19.5007) (82.0539, 19.6687) (81.7475, 19.7379) knots 0 0 0 1 2 2 2
  spline S119 degree 2 poles (81.7475, 19.7379) (81.5843, 19.7824) (81.0851, 19.8764) (80.8923, 19.9357) knots 0 0 0 1 2 2 2
  spline S120 degree 2 poles (80.8923, 19.9357) (80.3485, 20.1038) (79.8048, 20.7612) (79.8048, 21.3) knots 0 0 0 1 2 2 2
  spline S121 degree 2 poles (79.8048, 21.3) (79.8048, 21.6065) (80.0865, 22.1503) (80.3633, 22.3628) knots 0 0 0 1 2 2 2
  spline S122 degree 2 poles (80.3633, 22.3628) (80.6352, 22.5704) (81.441, 22.8176) (81.9501, 22.8176) knots 0 0 0 1 2 2 2
  spline S123 degree 2 poles (81.9501, 22.8176) (82.4346, 22.8176) (83.2453, 22.6248) (83.5221, 22.4914) knots 0 0 0 1 2 2 2
  line L129 (83.5221, 22.4914) -> (83.5221, 21.3247)
  line L130 (83.5221, 21.3247) -> (83.4084, 21.3247)
  spline S124 degree 2 poles (83.4084, 21.3247) (83.3343, 21.3841) (83.0129, 21.5768) (82.8646, 21.6461) knots 0 0 0 1 2 2 2
  spline S125 degree 2 poles (82.8646, 21.6461) (82.6817, 21.7251) (82.2369, 21.8339) (82.0045, 21.8339) knots 0 0 0 1 2 2 2
  spline S126 degree 2 poles (82.0045, 21.8339) (81.6931, 21.8339) (81.263, 21.6213) (81.263, 21.4483) knots 0 0 0 1 2 2 2
  spline S127 degree 2 poles (81.263, 21.4483) (81.263, 21.2901) (81.4756, 21.1122) (81.8315, 21.0232) knots 0 0 0 1 2 2 2
  spline S128 degree 2 poles (81.8315, 21.0232) (82.0144, 20.9787) (82.4939, 20.8947) (82.7163, 20.8205) knots 0 0 0 1 2 2 2
  spline S129 degree 2 poles (82.7163, 20.8205) (83.2107, 20.6623) (83.7248, 20.0444) (83.7248, 19.5303) knots 0 0 0 1 2 2 2
  spline S130 degree 2 poles (83.7248, 19.5303) (83.7248, 19.209) (83.4232, 18.6208) (83.1415, 18.423) knots 0 0 0 1 2 2 2
  spline S131 degree 2 poles (83.1415, 18.423) (82.8498, 18.2055) (82.049, 17.9683) (81.4904, 17.9683) knots 0 0 0 1 2 2 2
  line L131 (42.8563, 8.0483) -> (39.5739, 8.0483)
  line L132 (39.5739, 8.0483) -> (39.5739, 9.1112)
  line L133 (39.5739, 9.1112) -> (40.4489, 9.1112)
  line L134 (40.4489, 9.1112) -> (40.4489, 13.0855)
  line L135 (40.4489, 13.0855) -> (39.5739, 13.0855)
  line L136 (39.5739, 13.0855) -> (39.5739, 14.1483)
  line L137 (39.5739, 14.1483) -> (42.8563, 14.1483)
  line L138 (42.8563, 14.1483) -> (42.8563, 13.0855)
  line L139 (42.8563, 13.0855) -> (41.9813, 13.0855)
  line L140 (41.9813, 13.0855) -> (41.9813, 9.1112)
  line L141 (41.9813, 9.1112) -> (42.8563, 9.1112)
  line L142 (42.8563, 9.1112) -> (42.8563, 8.0483)
  line L143 (48.0961, 8.0483) -> (46.6527, 8.0483)
  line L144 (46.6527, 8.0483) -> (46.6527, 10.3272)
  spline S132 degree 2 poles (46.6527, 10.3272) (46.6527, 10.609) (46.6082, 11.1626) (46.5489, 11.2911) knots 0 0 0 1 2 2 2
  spline S133 degree 2 poles (46.5489, 11.2911) (46.4747, 11.4493) (46.1979, 11.5828) (45.9606, 11.5828) knots 0 0 0 1 2 2 2
  spline S134 degree 2 poles (45.9606, 11.5828) (45.7876, 11.5828) (45.4268, 11.4493) (45.2241, 11.306) knots 0 0 0 1 2 2 2
  line L145 (45.2241, 11.306) -> (45.2241, 8.0483)
  line L146 (45.2241, 8.0483) -> (43.7905, 8.0483)
  line L147 (43.7905, 8.0483) -> (43.7905, 12.6505)
  line L148 (43.7905, 12.6505) -> (45.2241, 12.6505)
  line L149 (45.2241, 12.6505) -> (45.2241, 12.1414)
  spline S135 degree 2 poles (45.2241, 12.1414) (45.5751, 12.438) (46.2424, 12.7741) (46.6478, 12.7741) knots 0 0 0 1 2 2 2
  spline S136 degree 2 poles (46.6478, 12.7741) (47.3497, 12.7741) (48.0961, 11.8843) (48.0961, 11.044) knots 0 0 0 1 2 2 2
  line L150 (48.0961, 11.044) -> (48.0961, 8.0483)
  line L151 (53.3409, 8.0483) -> (51.9074, 8.0483)
  line L152 (51.9074, 8.0483) -> (51.9074, 8.5278)
  spline S137 degree 2 poles (51.9074, 8.5278) (51.769, 8.4142) (51.4131, 8.1522) (51.2747, 8.083) knots 0 0 0 1 2 2 2
  spline S138 degree 2 poles (51.2747, 8.083) (51.1066, 8.0039) (50.7704, 7.9198) (50.5381, 7.9198) knots 0 0 0 1 2 2 2
  spline S139 degree 2 poles (50.5381, 7.9198) (49.7521, 7.9198) (48.8327, 9.2248) (48.8327, 10.3124) knots 0 0 0 1 2 2 2
  spline S140 degree 2 poles (48.8327, 10.3124) (48.8327, 10.9154) (49.1441, 11.8003) (49.416, 12.1265) knots 0 0 0 1 2 2 2
  spline S141 degree 2 poles (49.416, 12.1265) (49.6681, 12.4281) (50.3799, 12.7741) (50.7754, 12.7741) knots 0 0 0 1 2 2 2
  spline S142 degree 2 poles (50.7754, 12.7741) (51.1362, 12.7741) (51.6009, 12.6209) (51.9074, 12.4627) knots 0 0 0 1 2 2 2
  line L153 (51.9074, 12.4627) -> (51.9074, 14.4202)
  line L154 (51.9074, 14.4202) -> (53.3409, 14.4202)
  line L155 (53.3409, 14.4202) -> (53.3409, 8.0483)
  line L156 (51.9074, 9.3138) -> (51.9074, 11.5729)
  spline S143 degree 2 poles (51.9074, 11.5729) (51.8036, 11.6273) (51.4576, 11.6965) (51.334, 11.6965) knots 0 0 0 1 2 2 2
  spline S144 degree 2 poles (51.334, 11.6965) (50.8199, 11.6965) (50.3008, 10.9748) (50.3008, 10.3272) knots 0 0 0 1 2 2 2
  spline S145 degree 2 poles (50.3008, 10.3272) (50.3008, 9.645) (50.7161, 9.037) (51.1758, 9.037) knots 0 0 0 1 2 2 2
  spline S146 degree 2 poles (51.1758, 9.037) (51.3636, 9.037) (51.7492, 9.1853) (51.9074, 9.3138) knots 0 0 0 1 2 2 2
  spline S147 degree 2 poles (58.8527, 10.347) (58.8527, 9.21) (57.6119, 7.905) (56.4799, 7.905) knots 0 0 0 1 2 2 2